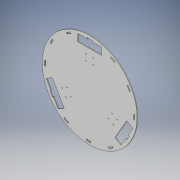
# Autodesk Inventor part: denew
Saved by Autodesk Inventor 2019 (Build 230136000, 136)
## iProperties
Created: 2021-01-20
Part Number: denew
Material: Generic
Document SubType Name: Modeling
Designer: Admin
Density: 1 g/cm^3
Appearance: Default
Author: Admin
Autodesk Inventor part; units mm, degrees
ref_plane "YZ Plane" through (0, 0, 0) normal (1, 0, 0) x (0, 1, 0)
ref_plane "XZ Plane" through (0, 0, 0) normal (0, 1, 0) x (-1, 0, 0)
ref_plane "XY Plane" through (0, 0, 0) normal (0, 0, 1) x (1, 0, 0)
sketch "Sketch1" plane through (0, 0, 0) normal (0, 0, 1) x (1, 0, 0)
  circle A0 centre (0, 0) radius 200
  line L0 (90.6699, 167.0448) -> (88.1699, 162.7147)
  line L1 (96.8301, 157.7147) -> (99.3301, 162.0448)
  line L2 (162.0448, 99.3301) -> (157.7147, 96.8301)
  line L3 (162.7147, 88.1699) -> (167.0448, 90.6699)
  line L4 (185, 5) -> (190, 5)
  line L5 (190, -5) -> (185, -5)
  line L6 (88.1699, -162.7147) -> (96.8301, -157.7147)
  line L7 (99.3301, -162.0448) -> (90.6699, -167.0448)
  line L8 (-5, -190) -> (-5, -185)
  line L9 (5, -185) -> (5, -190)
  line L10 (-99.3301, -162.0448) -> (-90.6699, -167.0448)
  line L11 (-88.1699, -162.7147) -> (-96.8301, -157.7147)
  line L12 (-190, 5) -> (-190, -5)
  line L13 (-190, -5) -> (-185, -5)
  line L14 (-185, -5) -> (-185, 5)
  line L15 (-167.0448, 90.6699) -> (-162.0448, 99.3301)
  line L16 (-157.7147, 96.8301) -> (-162.7147, 88.1699)
  line L17 (-99.3301, 162.0448) -> (-90.6699, 167.0448)
  line L18 (-88.1699, 162.7147) -> (-96.8301, 157.7147)
  line L19 (-190, -5) -> (-190, 5)
  line L20 (-185, 5) -> (-185, -5)
  line L21 (88.1699, 162.7147) -> (96.8301, 157.7147)
  line L22 (99.3301, 162.0448) -> (90.6699, 167.0448)
  line L23 (162.7147, 88.1699) -> (157.7147, 96.8301)
  line L24 (162.0448, 99.3301) -> (167.0448, 90.6699)
  line L25 (185, 5) -> (185, -5)
  line L26 (190, 5) -> (190, -5)
  line L27 (96.8301, -157.7147) -> (99.3301, -162.0448)
  line L28 (88.1699, -162.7147) -> (90.6699, -167.0448)
  line L29 (-5, -185) -> (5, -185)
  line L30 (-5, -190) -> (5, -190)
  line L31 (-99.3301, -162.0448) -> (-96.8301, -157.7147)
  line L32 (-90.6699, -167.0448) -> (-88.1699, -162.7147)
  line L33 (-190, 5) -> (-185, 5)
  line L34 (-162.0448, 99.3301) -> (-157.7147, 96.8301)
  line L35 (-167.0448, 90.6699) -> (-162.7147, 88.1699)
  line L36 (-99.3301, 162.0448) -> (-96.8301, 157.7147)
  line L37 (-90.6699, 167.0448) -> (-88.1699, 162.7147)
  line L38 (50, 182.5) -> (10, 182.5)
  line L39 (10, 182.5) -> (10, 187.5)
  line L40 (10, 187.5) -> (0, 187.5)
  line L41 (157.7147, 96.8301) -> (162.0448, 99.3301)
  line L42 (167.0448, 90.6699) -> (162.7147, 88.1699)
  line L43 (-99.3301, -162.0448) -> (-96.8301, -157.7147)
  line L44 (-88.1699, -162.7147) -> (-90.6699, -167.0448)
  line L45 (-99.3301, -162.0448) -> (-96.8301, -157.7147)
  line L46 (-88.1699, -162.7147) -> (-90.6699, -167.0448)
  line L47 (-99.3301, -162.0448) -> (-90.6699, -167.0448)
  circle A1 centre (14.945, 125) radius 1.73
  circle A2 centre (14.945, 100.94) radius 1.73
  circle A3 centre (-14.945, 100.94) radius 1.73
  circle A4 centre (-14.945, 125) radius 1.73
  circle A5 centre (-100.7807, -75.4427) radius 1.73
  circle A6 centre (-115.7257, -49.5573) radius 1.73
  circle A7 centre (-79.9441, -63.4127) radius 1.73
  circle A8 centre (-94.8891, -37.5273) radius 1.73
  circle A9 centre (115.7257, -49.5573) radius 1.73
  circle A10 centre (100.7807, -75.4427) radius 1.73
  circle A11 centre (94.8891, -37.5273) radius 1.73
  circle A12 centre (79.9441, -63.4127) radius 1.73
  line L48 (0, 152.5) -> (50, 152.5)
  line L49 (50, 152.5) -> (50, 182.5)
  line L50 (-10, 182.5) -> (-10, 187.5)
  line L51 (-10, 187.5) -> (0, 187.5)
  line L52 (-50, 182.5) -> (-10, 182.5)
  line L53 (0, 152.5) -> (-50, 152.5)
  line L54 (-50, 152.5) -> (-50, 182.5)
  circle A13 centre (0, 0) radius 200
  line L55 (-163.0496, -82.5897) -> (-167.3798, -85.0897)
  line L56 (-167.3798, -85.0897) -> (-162.3798, -93.75)
  line L57 (-183.0496, -47.9487) -> (-163.0496, -82.5897)
  line L58 (-132.0689, -76.25) -> (-157.0689, -32.9487)
  line L59 (-157.0689, -32.9487) -> (-183.0496, -47.9487)
  line L60 (-132.0689, -76.25) -> (-107.0689, -119.5513)
  line L61 (-157.3798, -102.4103) -> (-162.3798, -93.75)
  line L62 (-153.0496, -99.9103) -> (-157.3798, -102.4103)
  line L63 (-133.0496, -134.5513) -> (-153.0496, -99.9103)
  line L64 (-107.0689, -119.5513) -> (-133.0496, -134.5513)
  circle A14 centre (0, 0) radius 200
  line L65 (153.0496, -99.9103) -> (157.3798, -102.4103)
  line L66 (157.3798, -102.4103) -> (162.3798, -93.75)
  line L67 (133.0496, -134.5513) -> (153.0496, -99.9103)
  line L68 (132.0689, -76.25) -> (107.0689, -119.5513)
  line L69 (107.0689, -119.5513) -> (133.0496, -134.5513)
  line L70 (132.0689, -76.25) -> (157.0689, -32.9487)
  line L71 (167.3798, -85.0897) -> (162.3798, -93.75)
  line L72 (163.0496, -82.5897) -> (167.3798, -85.0897)
  line L73 (183.0496, -47.9487) -> (163.0496, -82.5897)
  line L74 (157.0689, -32.9487) -> (183.0496, -47.9487)
  dimension "d6" = 40
  dimension "d8" = 3.46
  dimension "d9" = 360
  dimension "d11" = 50
  dimension "d14" = 360
  constraints: 150 end point, 15 centre point, 11 equal length, 9 perpendicular, 3 vertical, 2 coincident, 2 horizontal, 2 point on line, 90 other
  measures "d6" distance of L38.start L39.start
  measures "d8" diameter of A1
  measures "d11" distance of L48.start L48.end
extrude "Extrusion1" add sketch "Sketch1" along normal blind 3
sketch "Sketch2" plane through (0, 0, 3) normal (0, 0, 1) x (1, 0, 0)
  line L0 (99.3301, 162.0448) -> (96.8301, 157.7147) projected
  line L1 (99.3301, 162.0448) -> (107.9904, 157.0448)
  line L2 (99.3301, 162.0448) -> (109.3301, 162.0448) construction
  line L3 (107.9904, 157.0448) -> (105.4904, 152.7147)
  line L4 (105.4904, 152.7147) -> (96.8301, 157.7147)
  circle A0 centre (0, 0) radius 200
  line L5 (96.8301, 157.7147) -> (99.3301, 162.0448)
  line L6 (5, 190) -> (15, 190)
  line L7 (5, 190) -> (13.6603, 195) construction
  line L8 (15, 190) -> (15, 185)
  line L9 (15, 185) -> (5, 185)
  line L10 (5, 185) -> (5, 190)
  line L11 (-90.6699, 167.0448) -> (-82.0096, 172.0448)
  line L12 (-90.6699, 167.0448) -> (-85.6699, 175.7051) construction
  line L13 (-82.0096, 172.0448) -> (-79.5096, 167.7147)
  line L14 (-79.5096, 167.7147) -> (-88.1699, 162.7147)
  line L15 (-88.1699, 162.7147) -> (-90.6699, 167.0448)
  line L16 (-162.0448, 99.3301) -> (-157.0448, 107.9904)
  line L17 (-162.0448, 99.3301) -> (-162.0448, 109.3301) construction
  line L18 (-157.0448, 107.9904) -> (-152.7147, 105.4904)
  line L19 (-152.7147, 105.4904) -> (-157.7147, 96.8301)
  line L20 (-157.7147, 96.8301) -> (-162.0448, 99.3301)
  line L21 (-190, 5) -> (-190, 15)
  line L22 (-190, 5) -> (-195, 13.6603) construction
  line L23 (-190, 15) -> (-185, 15)
  line L24 (-185, 15) -> (-185, 5)
  line L25 (-185, 5) -> (-190, 5)
  line L26 (-167.0448, -90.6699) -> (-172.0448, -82.0096)
  line L27 (-167.0448, -90.6699) -> (-175.7051, -85.6699) construction
  line L28 (-172.0448, -82.0096) -> (-167.7147, -79.5096)
  line L29 (-167.7147, -79.5096) -> (-162.7147, -88.1699)
  line L30 (-162.7147, -88.1699) -> (-167.0448, -90.6699)
  line L31 (-99.3301, -162.0448) -> (-107.9904, -157.0448)
  line L32 (-99.3301, -162.0448) -> (-109.3301, -162.0448) construction
  line L33 (-107.9904, -157.0448) -> (-105.4904, -152.7147)
  line L34 (-105.4904, -152.7147) -> (-96.8301, -157.7147)
  line L35 (-96.8301, -157.7147) -> (-99.3301, -162.0448)
  line L36 (-5, -190) -> (-15, -190)
  line L37 (-5, -190) -> (-13.6603, -195) construction
  line L38 (-15, -190) -> (-15, -185)
  line L39 (-15, -185) -> (-5, -185)
  line L40 (-5, -185) -> (-5, -190)
  line L41 (90.6699, -167.0448) -> (82.0096, -172.0448)
  line L42 (90.6699, -167.0448) -> (85.6699, -175.7051) construction
  line L43 (82.0096, -172.0448) -> (79.5096, -167.7147)
  line L44 (79.5096, -167.7147) -> (88.1699, -162.7147)
  line L45 (88.1699, -162.7147) -> (90.6699, -167.0448)
  line L46 (162.0448, -99.3301) -> (157.0448, -107.9904)
  line L47 (162.0448, -99.3301) -> (162.0448, -109.3301) construction
  line L48 (157.0448, -107.9904) -> (152.7147, -105.4904)
  line L49 (152.7147, -105.4904) -> (157.7147, -96.8301)
  line L50 (157.7147, -96.8301) -> (162.0448, -99.3301)
  line L51 (190, -5) -> (190, -15)
  line L52 (190, -5) -> (195, -13.6603) construction
  line L53 (190, -15) -> (185, -15)
  line L54 (185, -15) -> (185, -5)
  line L55 (185, -5) -> (190, -5)
  line L56 (167.0448, 90.6699) -> (172.0448, 82.0096)
  line L57 (167.0448, 90.6699) -> (175.7051, 85.6699) construction
  line L58 (172.0448, 82.0096) -> (167.7147, 79.5096)
  line L59 (167.7147, 79.5096) -> (162.7147, 88.1699)
  line L60 (162.7147, 88.1699) -> (167.0448, 90.6699)
  dimension "d18" = 10
  dimension "d19" = 30
  dimension "d22" = 360
  constraints: 120 end point, 3 perpendicular, 1 centre point, 1 coincident, 1 collinear, 1 equal length, 1 horizontal, 121 other
  measures "d18" distance of L0.start L1.end
  measures "d19" angle of L1 L2
extrude "Extrusion2" cut sketch "Sketch2" against normal blind 10 contours L1 L3 L4 L0 | L11 L13 L14 L15 | L16 L18 L19 L20 | L21 L23 L24 L25 | L31 L33 L34 L35 | L36 L38 L39 L40 | L41 L43 L44 L45 | L51 L53 L54 L55 | L56 L58 L59 L60
body "Solid1"
